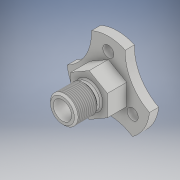
# Autodesk Inventor part: деталь из openedu
Saved by Autodesk Inventor 2019 (Build 230136000, 136)
## iProperties
Created: 2020-04-14
Part Number: деталь из openedu
Material: Типовые
Document SubType Name: Modeling
Designer: Антон
Density: 1 g/cm^3
Appearance: По умолчанию
Mass: 61.7919 g
Surface Area: 218.23 cm^2
Volume: 61.7919 cm^3
Author: Антон
Autodesk Inventor part; units mm, degrees
ref_plane "YZ Plane" through (0, 0, 0) normal (1, 0, 0) x (0, 1, 0)
ref_plane "XZ Plane" through (0, 0, 0) normal (0, 1, 0) x (-1, 0, 0)
ref_plane "XY Plane" through (0, 0, 0) normal (0, 0, 1) x (1, 0, 0)
sketch "Эскиз1" plane through (0, 0, 0) normal (0, 0, 1) x (1, 0, 0)
  circle A0 centre (0, 0) radius 45
  dimension "d0" = 90
  constraints: 1 centre point, 1 coincident
  measures "d0" diameter of A0
extrude "Выдавливание1" add sketch "Эскиз1" along normal blind 10
sketch "Эскиз2" plane through (0, 0, 10) normal (0, 0, 1) x (1, 0, 0)
  circle A0 centre (0, -77.7948) radius 49
  circle A1 centre (67.3723, 38.8974) radius 49
  circle A2 centre (-67.3723, 38.8974) radius 49
  point P0 (0, 0)
  dimension "d3" = 98
  dimension "d6" = 360
  constraints: 3 centre point, 1 vertical alignment, 7 other
  measures "d3" diameter of A0
extrude "Выдавливание2" cut sketch "Эскиз2" against normal blind 10
sketch "Эскиз3" plane through (0, 0, 10) normal (0, 0, 1) x (1, 0, 0)
  circle A0 centre (0, 30.6206) radius 6
  circle A1 centre (-26.5182, -15.3103) radius 6
  circle A2 centre (26.5182, -15.3103) radius 6
  point P0 (0, 0)
  dimension "d10" = 12
  dimension "d13" = 360
  constraints: 3 centre point, 1 vertical alignment, 7 other
  measures "d10" diameter of A0
hole "Отверстие1" at (0, 30.6206, 10) at (-26.5182, -15.3103, 10) at (26.5182, -15.3103, 10) direction (0, 0, -1) diameter 12 end through all
sketch "Эскиз4" plane through (0, 0, 10) normal (0, 0, 1) x (1, 0, 0)
  line L0 (-19.9186, -11.5) -> (-19.9186, 11.5)
  line L1 (-19.9186, 11.5) -> (0, 23)
  line L2 (0, 23) -> (19.9186, 11.5)
  line L3 (19.9186, 11.5) -> (19.9186, -11.5)
  line L4 (19.9186, -11.5) -> (0, -23)
  line L5 (0, -23) -> (-19.9186, -11.5)
  point P0 (0, 0)
  point P1 (0, 0)
  dimension "d22" = 46
  constraints: 12 end point, 1 coincident, 1 vertical alignment, 13 other
  measures "d22" distance of L4.end L1.end
extrude "Выдавливание3" add sketch "Эскиз4" along normal blind 21
hole "Отверстие2" at (0, 0, 0) direction (0, 0, 1) diameter 30 depth 25
chamfer "Фаска2" distance 4 angle 45 1 edges at (0, -15, 0) measured on face at (0, -15.5, 0)
sketch "Эскиз7" plane through (19.9186, -11.5, 10) normal (1, 0, 0) x (0, 0, -1)
  point P0 (10, 11.5)
sketch "Эскиз8" plane through (19.9186, -11.5, 10) normal (1, 0, 0) x (0, 0, -1)
  point P0 (10, 11.5)
sketch "Эскиз9" plane through (0, 0, 0) normal (1, 0, 0) x (0, 1, 0)
  point P0 (0, 0)
sketch "Эскиз10" plane through (0, 0, 0) normal (1, 0, 0) x (0, 1, 0)
  point P0 (0, 0)
sketch "Эскиз13" plane through (0, 0, 0) normal (1, 0, 0) x (0, 1, 0)
  line L0 (0, -6.2) -> (0, 37.2) projected
  line L1 (11.5, 31) -> (-11.5, 31) projected
  line L2 (-11.5, 31) -> (-23, 31) projected
  line L3 (-23, 31) -> (-11.5, 31) projected
  line L4 (-11.5, 31) -> (11.5, 31) projected
  line L5 (11.5, 31) -> (23, 31) projected
  line L6 (23, 31) -> (11.5, 31) projected
  line L7 (13.5, 31) -> (0, 31)
  line L8 (-11.5, 31) -> (11.5, 31) projected
  point P0 (0, 0)
  point P1 (0, 31)
  point P2 (0, 31)
  point P3 (0, 31)
  constraints: 3 midpoint, 2 end point, 1 coincident, 1 horizontal alignment
sketch "Эскиз14" plane through (0, 0, 0) normal (1, 0, 0) x (0, 1, 0)
  line L0 (0, 60) -> (15, 60)
  line L1 (15, 60) -> (15, 37.5)
  line L2 (15, 37.5) -> (13.5, 36)
  line L3 (13.5, 36) -> (13.5, 31)
  line L4 (13.5, 31) -> (0, 31)
  line L5 (0, 31) -> (0, 60)
  line L6 (-11.5, 31) -> (11.5, 31) projected
  point P0 (0, 0)
  dimension "d86" = 45
  dimension "d87" = 29
  dimension "d88" = 30
  dimension "d89" = 27
  dimension "d90" = 5
  constraints: 12 end point, 2 midpoint, 2 perpendicular, 1 horizontal, 1 horizontal alignment, 1 parallel, 1 vertical, 1 vertical alignment
  measures "d86" angle of L1 L2
  measures "d87" distance of L4.end L0.start
  measures "d88" diameter of L1 L5
  measures "d89" diameter of L3 L5
  measures "d90" distance of L2.end L3.end
revolve "Вращение2" add sketch "Эскиз14" angle 360 about axis through (0, 0, 31) along (0, 0, 1)
fillet "Сопряжение3" radius 0.5 1 edges at (0, -13.5, 36)
fillet "Сопряжение3" radius 1.6 1 edges at (0, -13.5, 31)
thread "Резьба3" size "M30x2" class "6g" standard "ISO Metric profile" full length
sketch "Эскиз15" plane through (0, 0, 60) normal (0, 0, 1) x (1, 0, 0)
  point P0 (0, 0)
hole "Отверстие5" at (0, 0, 60) direction (0, 0, -1) diameter 20 depth 40
chamfer "Фаска4" distance 2 angle 45 1 edges at (0, -15, 60)
